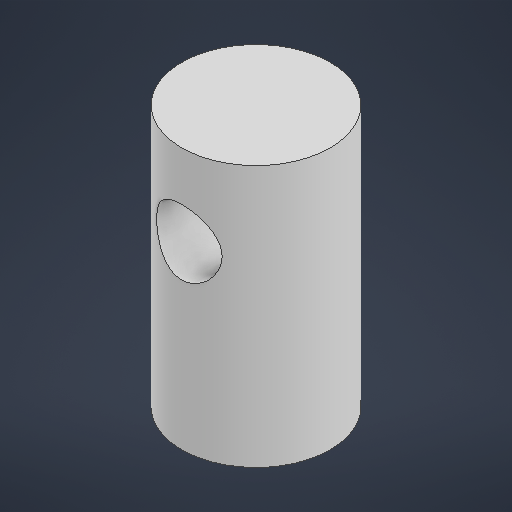
# Autodesk Inventor part: Lower_Chassis_Pin_1
Saved by Autodesk Inventor 2025.1 (Build 291241000, 241)
## iProperties
Created: 2024-08-04
Part Number: Lower_Chassis_Pin_1
Material: Generic
Document SubType Name: Modeling
Designer: Garfieldcmix
Density: 1 g/cm^3
Appearance: Default
Author: Garfieldcmix
Autodesk Inventor part; units mm, degrees
ref_plane "YZ Plane" through (0, 0, 0) normal (1, 0, 0) x (0, 1, 0)
ref_plane "XZ Plane" through (0, 0, 0) normal (0, 1, 0) x (-1, 0, 0)
sketch "Sketch1" plane through (0, 0, 0) normal (0, 1, 0) x (-1, 0, 0)
  circle A0 centre (0, 0) radius 2.4
  dimension "d0" = 4.8
  constraints: 1 centre point, 1 coincident
  measures "d0" diameter of A0
extrude "Extrusion1" add sketch "Sketch1" along normal blind 8
ref_plane "Work Plane1" through (0, 0, 2.4) normal (0, 0, 1) x (1, 0, 0)
sketch "Sketch2" plane through (0, 0, 2.4) normal (0, 0, 1) x (1, 0, 0)
  line L0 (2.4, 8) -> (-2.4, 8) construction
  line L1 (0, 8) -> (0, 5.5) construction
  point P0 (0, 0)
  dimension "d3" = 2.5
  constraints: 2 end point, 1 coincident, 1 midpoint, 1 perpendicular
  measures "d3" distance of L1.start L1.end
hole "Hole1" at (0, 5.5, 2.4) direction (0, 0, -1) diameter 2 end through all
offset faces "Size1" outward -0.13 faces at (-2.3689, 2.6667, -0.385)
body "Solid1"
